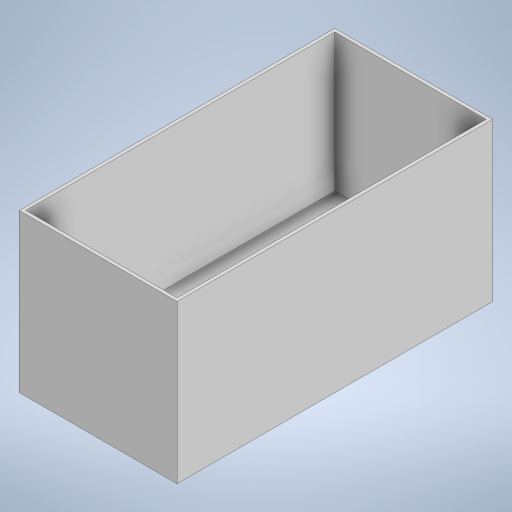
# Autodesk Inventor part: Cargo Container
Saved by Autodesk Inventor 2024 (Build 280153000, 153)
## iProperties
Created: 2023-11-13
Part Number: Cargo Container
Material: Generic
Document SubType Name: Modeling
Designer: Luke
Density: 1 g/cm^3
Appearance: Default
Author: Luke
Autodesk Inventor part; units mm, degrees
ref_plane "YZ Plane" through (0, 0, 0) normal (1, 0, 0) x (0, 1, 0)
ref_plane "XZ Plane" through (0, 0, 0) normal (0, 1, 0) x (-1, 0, 0)
ref_plane "XY Plane" through (0, 0, 0) normal (0, 0, 1) x (1, 0, 0)
sketch "Sketch1" plane through (0, 0, 0) normal (0, 1, 0) x (-1, 0, 0)
  line L0 (0, 0) -> (304.8, 0)
  line L1 (304.8, 0) -> (304.8, -609.6)
  line L2 (304.8, -609.6) -> (0, -609.6)
  line L3 (0, -609.6) -> (0, 0)
  dimension "d0" = 304.8
  dimension "d1" = 609.6
  constraints: 8 end point, 2 parallel, 1 horizontal, 1 perpendicular
  measures "d0" distance of L1.end L2.end
  measures "d1" distance between parallel lines of L2 L0
extrude "Extrusion1" add sketch "Sketch1" along normal blind 304.8
sketch "Sketch2" plane through (0, 304.8, 0) normal (0, 1, 0) x (1, 0, 0)
  line L0 (-298.45, 603.25) -> (-6.35, 603.25)
  line L1 (-6.35, 603.25) -> (-6.35, 6.35)
  line L2 (-6.35, 6.35) -> (-298.45, 6.35)
  line L3 (-298.45, 6.35) -> (-298.45, 603.25)
  line L4 (0, 0) -> (0, 609.6) projected
  line L5 (-304.8, 609.6) -> (-304.8, 0) projected
  line L6 (-304.8, 0) -> (0, 0) projected
  line L7 (0, 609.6) -> (-304.8, 609.6) projected
  dimension "d4" = 6.35
  dimension "d5" = 6.35
  dimension "d6" = 6.35
  dimension "d7" = 6.35
  constraints: 8 end point, 2 parallel, 1 horizontal, 1 perpendicular
  measures "d4" distance between parallel lines of L4 L1
  measures "d5" distance between parallel lines of L5 L3
  measures "d6" distance between parallel lines of L6 L2
  measures "d7" distance between parallel lines of L7 L0
extrude "Extrusion2" cut sketch "Sketch2" against normal blind 266.7 contours L0 L1 L2 L3
sketch "Sketch3" plane through (0, 0, 0) normal (0, -1, 0) x (1, 0, 0)
  line L0 (-298.45, -6.35) -> (-298.45, -603.25) projected
  line L1 (-6.35, -6.35) -> (-298.45, -6.35)
  line L2 (-298.45, -6.35) -> (-298.45, -603.25)
  line L3 (-298.45, -603.25) -> (-6.35, -603.25)
  line L4 (-6.35, -603.25) -> (-6.35, -6.35)
  line L5 (0, 0) -> (0, -609.6) projected
  line L6 (-304.8, 0) -> (0, 0) projected
  dimension "d10" = 6.35
  dimension "d11" = 6.35
  constraints: 8 end point, 2 parallel, 1 horizontal, 1 perpendicular
  measures "d10" distance between parallel lines of L5 L4
  measures "d11" distance between parallel lines of L6 L1
extrude "Extrusion3" cut sketch "Sketch3" against normal blind 31.75
body "Solid1"
